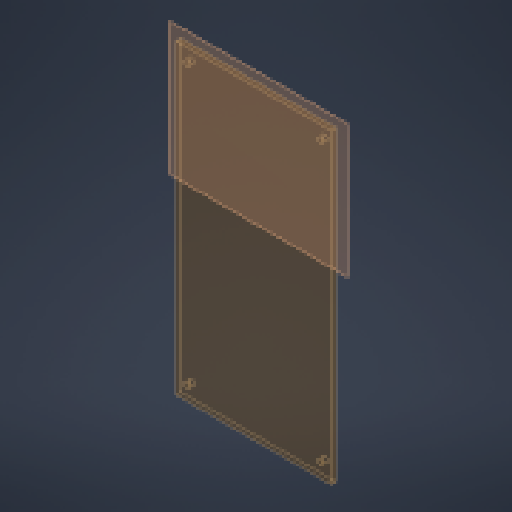
# Autodesk Inventor part: BP_CoverPlateAcrylic
Saved by Autodesk Inventor 2026.1 (Build 301233020, 233B)
## iProperties
Created: 2025-09-13
Part Number: BP_CoverPlateAcrylic
Material: PMMA Plastic
Document SubType Name: Modeling
Designer: atrus
Density: 1.188 g/cm^3
Appearance: Polycarbonate - Smoked
Author: atrus
Autodesk Inventor part; units mm, degrees
ref_plane "YZ Plane" through (0, 0, 0) normal (1, 0, 0) x (0, 1, 0)
ref_plane "XZ Plane" through (0, 0, 0) normal (0, 1, 0) x (-1, 0, 0)
ref_plane "XY Plane" through (0, 0, 0) normal (0, 0, 1) x (1, 0, 0)
ref_plane "Work Plane1" through (0, 0, 0) normal (0, 0, 1) x (1, 0, 0)
sketch "Sketch1" plane through (0, 0, 0) normal (0, 0, 1) x (1, 0, 0)
  line L0 (-10.216, 5.2) -> (85.116, 5.2)
  line L1 (85.116, 5.2) -> (85.116, -183)
  line L2 (85.116, -183) -> (-10.216, -183)
  line L3 (-10.216, -183) -> (-10.216, 5.2)
  line L4 (-8.95, -6.8) -> (0, -6.8)
  line L5 (-10.416, 5.4) -> (85.316, 5.4)
  circle A0 centre (78.4, -174.4) radius 1.9
  circle A1 centre (-3.5, -174.4) radius 1.9
  line L6 (85.316, -183.2) -> (85.316, -110.8)
  line L7 (85.316, -110.8) -> (83.85, -110.8)
  line L8 (74.9, -170.9) -> (74.9, -177.9)
  line L9 (83.85, -110.8) -> (83.85, -170.9)
  line L10 (83.85, -170.9) -> (74.9, -170.9)
  line L11 (0, -177.9) -> (74.9, -177.9)
  line L12 (0, -170.9) -> (0, -177.9)
  line L13 (0, -170.9) -> (-8.95, -170.9)
  line L14 (-8.95, -170.9) -> (-8.95, -110.8)
  line L15 (-8.95, -110.8) -> (-10.416, -110.8)
  line L16 (-10.416, -110.8) -> (-10.416, -183.2)
  line L17 (-10.416, -183.2) -> (85.316, -183.2)
  circle A2 centre (78.4, -174.4) radius 1.9
  circle A3 centre (-3.5, -174.4) radius 1.9
  line L18 (85.316, -183.2) -> (85.316, -110.8)
  line L19 (85.316, -110.8) -> (83.85, -110.8)
  line L20 (74.9, -170.9) -> (74.9, -177.9)
  line L21 (83.85, -110.8) -> (83.85, -170.9)
  line L22 (83.85, -170.9) -> (74.9, -170.9)
  line L23 (0, -177.9) -> (74.9, -177.9)
  line L24 (0, -170.9) -> (0, -177.9)
  line L25 (0, -170.9) -> (-8.95, -170.9)
  line L26 (-8.95, -170.9) -> (-8.95, -110.8)
  line L27 (-8.95, -110.8) -> (-10.416, -110.8)
  line L28 (-10.416, -110.8) -> (-10.416, -183.2)
  line L29 (-10.416, -183.2) -> (85.316, -183.2)
  line L30 (74.9, 0.2) -> (0, 0.2)
  line L31 (0, 0.2) -> (0, -6.8)
  line L32 (83.85, -6.8) -> (83.85, -67)
  line L33 (83.85, -67) -> (85.316, -67)
  line L34 (85.316, -67) -> (85.316, 5.4)
  line L35 (85.316, 5.4) -> (-10.416, 5.4)
  line L36 (-10.416, 5.4) -> (-10.416, -67)
  line L37 (-10.416, -67) -> (-8.95, -67)
  line L38 (-8.95, -67) -> (-8.95, -6.8)
  line L39 (-8.95, -6.8) -> (0, -6.8)
  line L40 (0, 0.2) -> (0, -6.8)
  line L41 (74.9, 0.2) -> (0, 0.2)
  line L42 (74.9, -6.8) -> (74.9, 0.2)
  line L43 (74.9, -6.8) -> (83.85, -6.8)
  circle A4 centre (78.4, -3.3) radius 1.9
  circle A5 centre (-3.5, -3.3) radius 1.9
  point P0 (0, 0)
extrude "Extrusion1" add sketch "Sketch1" along normal blind 3 contours L0 L1 L33 L32 L43 L42 L30 L31 L4 L38 L37 L3 | L37 L38 L4 L31 L30 L42 L43 L32 L33 L1 L7 L9 L10 L8 L11 L12 L13 L14 L15 L3 | L15 L14 L13 L12 L11 L8 L10 L9 L7 L1 L2 L3 | A0 | A1 | A4 | A5
sketch "Sketch2" plane through (0, 0, 3) normal (0, 0, 1) x (1, 0, 0)
  circle A0 centre (78.4, -3.3) radius 1.9 projected
  circle A1 centre (-3.5, -3.3) radius 1.9 projected
  circle A2 centre (78.4, -174.4) radius 1.9 projected
  circle A3 centre (-3.5, -174.4) radius 1.9 projected
  point P0 (0, 0)
extrude "Extrusion2" cut sketch "Sketch2" against normal blind 3
body "Solid1"
